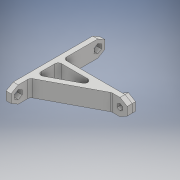
# Autodesk Inventor part: GPS_holder
Saved by Autodesk Inventor 2018 (Build 220112000, 112)
## iProperties
Created: 2018-07-16
Part Number: GPS_holder
Material: Generic
Document SubType Name: Modeling
Designer: Tsche
Density: 1 g/cm^3
Appearance: Default
Author: Tsche
Autodesk Inventor part; units mm, degrees
ref_plane "YZ Plane" through (0, 0, 0) normal (1, 0, 0) x (0, 1, 0)
ref_plane "XZ Plane" through (0, 0, 0) normal (0, 1, 0) x (-1, 0, 0)
ref_plane "XY Plane" through (0, 0, 0) normal (0, 0, 1) x (1, 0, 0)
sketch "Sketch1" plane through (0, 0, 0) normal (0, 0, 1) x (1, 0, 0)
  line L0 (3, -25) -> (44.33, -25)
  line L1 (44.33, -25) -> (44.33, -28)
  line L2 (44.33, -28) -> (35, -28)
  line L3 (35, -28) -> (3, -45)
  line L4 (3, -45) -> (3, -56.285)
  line L5 (3, -56.285) -> (0, -56.285)
  line L6 (0, -56.285) -> (0, 0)
  line L7 (3, -41.6029) -> (28.6055, -28)
  line L8 (28.6055, -28) -> (3, -28)
  line L9 (3, -41.6029) -> (3, -28)
  line L10 (0, -4.33) -> (3, -4.33) construction
  line L11 (0, -2.08) -> (3, -2.08) construction
  line L12 (0, -6.58) -> (3, -6.58) construction
  line L13 (0, -51.955) -> (3, -51.955) construction
  line L14 (0, -49.705) -> (3, -49.705) construction
  line L15 (0, -54.205) -> (3, -54.205) construction
  line L16 (40, -25) -> (40, -28) construction
  line L17 (0, 0) -> (3, 0)
  line L18 (3, 0) -> (3, -25)
  dimension "d1" = 3
  dimension "d2" = 3
  dimension "d3" = 3
  dimension "d6" = 20
  dimension "d8" = 4.5
  dimension "d13" = 47.625
  dimension "d18" = 40
  dimension "d48" = 4.33
  dimension "d49" = 5
  dimension "d55" = 4.33
  dimension "d56" = 25
  dimension "d59" = 4.33
  constraints: 38 end point, 12 point on line, 10 perpendicular, 2 horizontal, 2 parallel, 1 collinear, 1 vertical, 10 other
  measures "d1" distance between parallel lines of L0 L2
  measures "d2" distance of L4.end L5.end
  measures "d3" distance between parallel lines of L3 L7
  measures "d6" distance from line of L0 L3.end
  measures "d8" distance between parallel lines of L11 L12
  measures "d13" distance of L10.end L13.end
  measures "d18" distance between parallel lines of L6 L16
  measures "d48" distance between parallel lines of L1 L16
  measures "d49" distance from line of L2.end L16
  measures "d55" distance between parallel lines of L17 L10
  measures "d56" distance between parallel lines of L17 L0
  measures "d59" distance between parallel lines of L13 L5
extrude "Extrusion1" add sketch "Sketch1" along normal mid plane 10
fillet "Fillet2" radius 2 6 edges at (3, -45, 0) (35, -28, 0) (28.6055, -28, 0) (3, -41.6029, 0) (3, -28, 0) (3, -25, 0)
sketch "Sketch3" plane through (0, -56.285, 5) normal (-1, 0, 0) x (0, 0, 1)
  line L0 (-2.4019, 51.955) -> (-3.701, 49.705)
  line L1 (-3.701, 49.705) -> (-6.299, 49.705)
  line L2 (-6.299, 49.705) -> (-7.5981, 51.955)
  line L3 (-7.5981, 51.955) -> (-6.299, 54.205)
  line L4 (-6.299, 54.205) -> (-3.701, 54.205)
  line L5 (-3.701, 54.205) -> (-2.4019, 51.955)
  line L6 (-6.299, 6.58) -> (-3.701, 6.58)
  line L7 (-3.701, 6.58) -> (-2.4019, 4.33)
  line L8 (-2.4019, 4.33) -> (-3.701, 2.08)
  line L9 (-3.701, 2.08) -> (-6.299, 2.08)
  line L10 (-6.299, 2.08) -> (-7.5981, 4.33)
  line L11 (-7.5981, 4.33) -> (-6.299, 6.58)
  point P0 (-5, 56.285)
  point P1 (-5, 51.955)
  point P2 (-5, 51.955)
  point P3 (-5, 4.33)
  point P4 (-5, 4.33)
  dimension "d60" = 4.5
  constraints: 24 end point, 2 coincident, 2 horizontal, 1 parallel, 26 other
  measures "d60" distance between parallel lines of L1 L4
extrude "Extrusion3" cut sketch "Sketch3" against normal through all
sketch "Sketch4" plane through (44.33, -25, 5) normal (0, 1, 0) x (1, 0, 0)
  line L0 (-39.33, 10) -> (0, 10) construction
  line L1 (-4.33, 10) -> (0.0001, 7.5)
  line L2 (0.0001, 7.5) -> (0.0001, 2.5)
  line L3 (0.0001, 2.5) -> (-4.33, 0)
  line L4 (-4.33, 0) -> (-8.6601, 2.5)
  line L5 (-8.6601, 2.5) -> (-8.6601, 7.5)
  line L6 (-8.6601, 7.5) -> (-4.33, 10)
  line L7 (-4.33, 6.9053) -> (-2.68, 5.9526)
  line L8 (-2.68, 5.9526) -> (-2.68, 4.0474)
  line L9 (-2.68, 4.0474) -> (-4.33, 3.0947)
  line L10 (-4.33, 3.0947) -> (-5.98, 4.0474)
  line L11 (-5.98, 4.0474) -> (-5.98, 5.9526)
  line L12 (-5.98, 5.9526) -> (-4.33, 6.9053)
  point P0 (-44.33, 5)
  point P1 (-4.33, 5)
  point P2 (-4.33, 5)
  point P3 (-4.33, 5)
  dimension "d63" = 3.3
  constraints: 24 end point, 2 coincident, 2 vertical, 1 point on line, 26 other
  measures "d63" distance between parallel lines of L8 L11
extrude "Extrusion4" add sketch "Sketch4" along normal blind 2
extrude "Extrusion5" cut sketch "Sketch4" against normal through all contours L7 L8 L9 L10 L11 L12
chamfer "Chamfer1" distance 2.5 angle 60 2 edges at (44.33, -26.5, 5) (44.33, -26.5, -5) measured on face at (44.33, -27, -0.8334)
chamfer "Chamfer2" distance 2.5 angle 60 2 edges at (1.5, 0, -5) (1.5, 0, 5) measured on face at (2, 0, -1.6667)
chamfer "Chamfer3" distance 2.5 angle 60 2 edges at (1.5, -56.285, 5) (1.5, -56.285, -5) measured on face at (2, -56.285, 1.6667)
body "Solid1"
